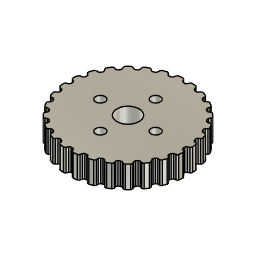
Timing Pulley Motor (Autodesk Fusion 360 design; units mm, degrees)
Autodesk Fusion 360 part; units mm, degrees
note: some values were not read from the file. Set by a fixed rule: which sketch regions a step uses.
(part 1 of 2)
sketch "スケッチ1" plane through (0, 0, 0) normal (0, 0, 1) x (1, 0, 0)
  circle A0 centre (0, 0) radius 4
  line L0 (-4, 0) -> (3, 0)
  line L1 (3, 2.6458) -> (3, -2.6458)
  circle A1 centre (0, 0) radius 20
  dimension "d1" = 8
  dimension "d2" = 7
  dimension "d3" = 40
  constraint coincident A0.centre A1.centre
  constraint coincident A0 L0.start
  constraint horizontal L0
  constraint coincident A0 L1.start
  constraint coincident A0 L1.end
  constraint perpendicular L0 L1
  measures "d1" diameter of A0
  measures "d2" distance of L0.start L0.end
  measures "d3" diameter of A1
extrude "押し出し1" add sketch "スケッチ1" along normal blind 8 contours A0 L1 | A0 L0 L1 | A0 L0 L1 | A1
sketch "スケッチ2" plane through (0, 0, 8) normal (0, 0, 1) x (-1, 0, 0)
  circle A0 centre (0, 0) radius 20
  circle A1 centre (0, 0) radius 22.635
  line L0 (0, 0) -> (22.635, 0)
  line L1 (0, 0) -> (22.0675, 5.0368)
  line L2 (0, 0) -> (20.3934, 9.821)
  line L3 (0, 0) -> (17.6968, 14.1127)
  line L4 (0, 0) -> (14.1127, 17.6968)
  line L5 (0, 0) -> (9.821, 20.3934)
  line L6 (0, 0) -> (5.0368, 22.0675)
  line L7 (0, 0) -> (0, 22.635)
  line L8 (0, 0) -> (-5.0368, 22.0675)
  line L9 (0, 0) -> (-9.821, 20.3934)
  line L10 (0, 0) -> (-14.1127, 17.6968)
  line L11 (0, 0) -> (-17.6968, 14.1127)
  line L12 (0, 0) -> (-20.3934, 9.821)
  line L13 (0, 0) -> (-22.0675, 5.0368)
  line L14 (0, 0) -> (-22.635, 0)
  line L15 (0, 0) -> (-22.0675, -5.0368)
  line L16 (0, 0) -> (-20.3934, -9.821)
  line L17 (0, 0) -> (-17.6968, -14.1127)
  line L18 (0, 0) -> (-14.1127, -17.6968)
  line L19 (0, 0) -> (-9.821, -20.3934)
  line L20 (0, 0) -> (-5.0368, -22.0675)
  line L21 (0, 0) -> (0, -22.635)
  line L22 (0, 0) -> (5.0368, -22.0675)
  line L23 (0, 0) -> (9.821, -20.3934)
  line L24 (0, 0) -> (14.1127, -17.6968)
  line L25 (0, 0) -> (17.6968, -14.1127)
  line L26 (0, 0) -> (20.3934, -9.821)
  line L27 (0, 0) -> (22.0675, -5.0368)
  line L28 (20.5872, -0.8492) -> (21.2144, -1.1417)
  line L29 (20.235, -0.685) -> (21.7353, -0.685) construction
  line L30 (20.5872, 0.8492) -> (21.2144, 1.1417)
  line L31 (20.235, 0.685) -> (21.7353, 0.685) construction
  arc A2 (20.235, -0.2964) -> (20.5872, -0.8492) centre (20.845, -0.2964) ccw
  arc A3 (20.5872, 0.8492) -> (20.235, 0.2964) centre (20.845, 0.2964) ccw
  arc A4 (21.5646, -1.7437) -> (21.2144, -1.1417) centre (20.9566, -1.6945) ccw
  arc A5 (21.2144, 1.1417) -> (21.5646, 1.7437) centre (20.9566, 1.6945) ccw
  arc A6 (21.412, 3.0986) -> (20.9366, 3.6076) centre (20.8082, 3.0112) ccw
  line L32 (20.26, 3.7531) -> (20.9366, 3.6076)
  arc A7 (19.7936, 4.2138) -> (20.26, 3.7531) centre (20.3883, 4.3495) ccw
  arc A8 (19.8821, 5.409) -> (19.6617, 4.7917) centre (20.2564, 4.9274) ccw
  line L33 (19.8821, 5.409) -> (20.4285, 5.8337)
  arc A9 (20.4285, 5.8337) -> (20.6359, 6.4986) centre (20.0541, 6.3153) ccw
  arc A10 (20.1856, 7.7855) -> (19.6089, 8.1759) centre (19.6165, 7.566) ccw
  line L34 (18.9169, 8.1673) -> (19.6089, 8.1759)
  arc A11 (18.3597, 8.5126) -> (18.9169, 8.1673) centre (18.9093, 8.7773) ccw
  arc A12 (18.18, 9.6976) -> (18.1025, 9.0467) centre (18.6521, 9.3113) ccw
  line L35 (18.18, 9.6976) -> (18.6181, 10.2332)
  arc A13 (18.6181, 10.2332) -> (18.6725, 10.9276) centre (18.146, 10.6195) ccw
  arc A14 (17.9471, 12.082) -> (17.2979, 12.3343) centre (17.4411, 11.7414) ccw
  line L36 (16.6252, 12.172) -> (17.2979, 12.3343)
  arc A15 (16.0052, 12.3846) -> (16.6252, 12.172) centre (16.4821, 12.7649) ccw
  arc A16 (15.5662, 13.4999) -> (15.6356, 12.848) centre (16.1125, 13.2284) ccw
  line L37 (15.5662, 13.4999) -> (15.8742, 14.1196)
  arc A17 (15.8742, 14.1196) -> (15.7727, 14.8086) centre (15.328, 14.3911) ccw
  arc A18 (14.8086, 15.7727) -> (14.1196, 15.8742) centre (14.3911, 15.328) ccw
  line L38 (13.4999, 15.5662) -> (14.1196, 15.8742)
  arc A19 (12.848, 15.6356) -> (13.4999, 15.5662) centre (13.2284, 16.1125) ccw
  arc A20 (12.172, 16.6252) -> (12.3846, 16.0052) centre (12.7649, 16.4821) ccw
  line L39 (12.172, 16.6252) -> (12.3343, 17.2979)
  arc A21 (12.3343, 17.2979) -> (12.082, 17.9471) centre (11.7414, 17.4411) ccw
  arc A22 (10.9276, 18.6725) -> (10.2332, 18.6181) centre (10.6195, 18.146) ccw
  line L40 (9.6976, 18.18) -> (10.2332, 18.6181)
  arc A23 (9.0467, 18.1025) -> (9.6976, 18.18) centre (9.3113, 18.6521) ccw
  arc A24 (8.1673, 18.9169) -> (8.5126, 18.3597) centre (8.7773, 18.9093) ccw
  line L41 (8.1673, 18.9169) -> (8.1759, 19.6089)
  arc A25 (8.1759, 19.6089) -> (7.7855, 20.1856) centre (7.566, 19.6165) ccw
  arc A26 (6.4986, 20.6359) -> (5.8337, 20.4285) centre (6.3153, 20.0541) ccw
  line L42 (5.409, 19.8821) -> (5.8337, 20.4285)
  arc A27 (4.7917, 19.6617) -> (5.409, 19.8821) centre (4.9274, 20.2564) ccw
  arc A28 (3.7531, 20.26) -> (4.2138, 19.7936) centre (4.3495, 20.3883) ccw
  line L43 (3.7531, 20.26) -> (3.6076, 20.9366)
  arc A29 (3.6076, 20.9366) -> (3.0986, 21.412) centre (3.0112, 20.8082) ccw
  arc A30 (1.7437, 21.5646) -> (1.1417, 21.2144) centre (1.6945, 20.9566) ccw
  line L44 (0.8492, 20.5872) -> (1.1417, 21.2144)
  arc A31 (0.2964, 20.235) -> (0.8492, 20.5872) centre (0.2964, 20.845) ccw
  arc A32 (-0.8492, 20.5872) -> (-0.2964, 20.235) centre (-0.2964, 20.845) ccw
  line L45 (-0.8492, 20.5872) -> (-1.1417, 21.2144)
  arc A33 (-1.1417, 21.2144) -> (-1.7437, 21.5646) centre (-1.6945, 20.9566) ccw
  arc A34 (-3.0986, 21.412) -> (-3.6076, 20.9366) centre (-3.0112, 20.8082) ccw
  line L46 (-3.7531, 20.26) -> (-3.6076, 20.9366)
  arc A35 (-4.2138, 19.7936) -> (-3.7531, 20.26) centre (-4.3495, 20.3883) ccw
  arc A36 (-5.409, 19.8821) -> (-4.7917, 19.6617) centre (-4.9274, 20.2564) ccw
  line L47 (-5.409, 19.8821) -> (-5.8337, 20.4285)
  arc A37 (-5.8337, 20.4285) -> (-6.4986, 20.6359) centre (-6.3153, 20.0541) ccw
  arc A38 (-7.7855, 20.1856) -> (-8.1759, 19.6089) centre (-7.566, 19.6165) ccw
  line L48 (-8.1673, 18.9169) -> (-8.1759, 19.6089)
  arc A39 (-8.5126, 18.3597) -> (-8.1673, 18.9169) centre (-8.7773, 18.9093) ccw
  arc A40 (-9.6976, 18.18) -> (-9.0467, 18.1025) centre (-9.3113, 18.6521) ccw
  line L49 (-9.6976, 18.18) -> (-10.2332, 18.6181)
  arc A41 (-10.2332, 18.6181) -> (-10.9276, 18.6725) centre (-10.6195, 18.146) ccw
  arc A42 (-12.082, 17.9471) -> (-12.3343, 17.2979) centre (-11.7414, 17.4411) ccw
  line L50 (-12.172, 16.6252) -> (-12.3343, 17.2979)
  arc A43 (-12.3846, 16.0052) -> (-12.172, 16.6252) centre (-12.7649, 16.4821) ccw
  arc A44 (-13.4999, 15.5662) -> (-12.848, 15.6356) centre (-13.2284, 16.1125) ccw
  line L51 (-13.4999, 15.5662) -> (-14.1196, 15.8742)
  arc A45 (-14.1196, 15.8742) -> (-14.8086, 15.7727) centre (-14.3911, 15.328) ccw
  arc A46 (-15.7727, 14.8086) -> (-15.8742, 14.1196) centre (-15.328, 14.3911) ccw
  line L52 (-15.5662, 13.4999) -> (-15.8742, 14.1196)
  arc A47 (-15.6356, 12.848) -> (-15.5662, 13.4999) centre (-16.1125, 13.2284) ccw
  arc A48 (-16.6252, 12.172) -> (-16.0052, 12.3846) centre (-16.4821, 12.7649) ccw
  line L53 (-16.6252, 12.172) -> (-17.2979, 12.3343)
  arc A49 (-17.2979, 12.3343) -> (-17.9471, 12.082) centre (-17.4411, 11.7414) ccw
  arc A50 (-18.6725, 10.9276) -> (-18.6181, 10.2332) centre (-18.146, 10.6195) ccw
  line L54 (-18.18, 9.6976) -> (-18.6181, 10.2332)
  arc A51 (-18.1025, 9.0467) -> (-18.18, 9.6976) centre (-18.6521, 9.3113) ccw
  arc A52 (-18.9169, 8.1673) -> (-18.3597, 8.5126) centre (-18.9093, 8.7773) ccw
  line L55 (-18.9169, 8.1673) -> (-19.6089, 8.1759)
  arc A53 (-19.6089, 8.1759) -> (-20.1856, 7.7855) centre (-19.6165, 7.566) ccw
  arc A54 (-20.6359, 6.4986) -> (-20.4285, 5.8337) centre (-20.0541, 6.3153) ccw
  line L56 (-19.8821, 5.409) -> (-20.4285, 5.8337)
  arc A55 (-19.6617, 4.7917) -> (-19.8821, 5.409) centre (-20.2564, 4.9274) ccw
  arc A56 (-20.26, 3.7531) -> (-19.7936, 4.2138) centre (-20.3883, 4.3495) ccw
  line L57 (-20.26, 3.7531) -> (-20.9366, 3.6076)
  arc A57 (-20.9366, 3.6076) -> (-21.412, 3.0986) centre (-20.8082, 3.0112) ccw
  arc A58 (-21.5646, 1.7437) -> (-21.2144, 1.1417) centre (-20.9566, 1.6945) ccw
  line L58 (-20.5872, 0.8492) -> (-21.2144, 1.1417)
  arc A59 (-20.235, 0.2964) -> (-20.5872, 0.8492) centre (-20.845, 0.2964) ccw
  arc A60 (-20.5872, -0.8492) -> (-20.235, -0.2964) centre (-20.845, -0.2964) ccw
  line L59 (-20.5872, -0.8492) -> (-21.2144, -1.1417)
  arc A61 (-21.2144, -1.1417) -> (-21.5646, -1.7437) centre (-20.9566, -1.6945) ccw
  arc A62 (-21.412, -3.0986) -> (-20.9366, -3.6076) centre (-20.8082, -3.0112) ccw
  line L60 (-20.26, -3.7531) -> (-20.9366, -3.6076)
  arc A63 (-19.7936, -4.2138) -> (-20.26, -3.7531) centre (-20.3883, -4.3495) ccw
  arc A64 (-19.8821, -5.409) -> (-19.6617, -4.7917) centre (-20.2564, -4.9274) ccw
  line L61 (-19.8821, -5.409) -> (-20.4285, -5.8337)
  arc A65 (-20.4285, -5.8337) -> (-20.6359, -6.4986) centre (-20.0541, -6.3153) ccw
  arc A66 (-20.1856, -7.7855) -> (-19.6089, -8.1759) centre (-19.6165, -7.566) ccw
  line L62 (-18.9169, -8.1673) -> (-19.6089, -8.1759)
  arc A67 (-18.3597, -8.5126) -> (-18.9169, -8.1673) centre (-18.9093, -8.7773) ccw
  arc A68 (-18.18, -9.6976) -> (-18.1025, -9.0467) centre (-18.6521, -9.3113) ccw
  line L63 (-18.18, -9.6976) -> (-18.6181, -10.2332)
  arc A69 (-18.6181, -10.2332) -> (-18.6725, -10.9276) centre (-18.146, -10.6195) ccw
  arc A70 (-17.9471, -12.082) -> (-17.2979, -12.3343) centre (-17.4411, -11.7414) ccw
  line L64 (-16.6252, -12.172) -> (-17.2979, -12.3343)
  arc A71 (-16.0052, -12.3846) -> (-16.6252, -12.172) centre (-16.4821, -12.7649) ccw
  arc A72 (-15.5662, -13.4999) -> (-15.6356, -12.848) centre (-16.1125, -13.2284) ccw
  line L65 (-15.5662, -13.4999) -> (-15.8742, -14.1196)
  arc A73 (-15.8742, -14.1196) -> (-15.7727, -14.8086) centre (-15.328, -14.3911) ccw
  arc A74 (-14.8086, -15.7727) -> (-14.1196, -15.8742) centre (-14.3911, -15.328) ccw
  line L66 (-13.4999, -15.5662) -> (-14.1196, -15.8742)
  arc A75 (-12.848, -15.6356) -> (-13.4999, -15.5662) centre (-13.2284, -16.1125) ccw
  arc A76 (-12.172, -16.6252) -> (-12.3846, -16.0052) centre (-12.7649, -16.4821) ccw
  line L67 (-12.172, -16.6252) -> (-12.3343, -17.2979)
  arc A77 (-12.3343, -17.2979) -> (-12.082, -17.9471) centre (-11.7414, -17.4411) ccw
  arc A78 (-10.9276, -18.6725) -> (-10.2332, -18.6181) centre (-10.6195, -18.146) ccw
  line L68 (-9.6976, -18.18) -> (-10.2332, -18.6181)
  arc A79 (-9.0467, -18.1025) -> (-9.6976, -18.18) centre (-9.3113, -18.6521) ccw
  arc A80 (-8.1673, -18.9169) -> (-8.5126, -18.3597) centre (-8.7773, -18.9093) ccw
  line L69 (-8.1673, -18.9169) -> (-8.1759, -19.6089)
  arc A81 (-8.1759, -19.6089) -> (-7.7855, -20.1856) centre (-7.566, -19.6165) ccw
  arc A82 (-6.4986, -20.6359) -> (-5.8337, -20.4285) centre (-6.3153, -20.0541) ccw
  line L70 (-5.409, -19.8821) -> (-5.8337, -20.4285)
  arc A83 (-4.7917, -19.6617) -> (-5.409, -19.8821) centre (-4.9274, -20.2564) ccw
  arc A84 (-3.7531, -20.26) -> (-4.2138, -19.7936) centre (-4.3495, -20.3883) ccw
  line L71 (-3.7531, -20.26) -> (-3.6076, -20.9366)
  arc A85 (-3.6076, -20.9366) -> (-3.0986, -21.412) centre (-3.0112, -20.8082) ccw
  arc A86 (-1.7437, -21.5646) -> (-1.1417, -21.2144) centre (-1.6945, -20.9566) ccw
  line L72 (-0.8492, -20.5872) -> (-1.1417, -21.2144)
  arc A87 (-0.2964, -20.235) -> (-0.8492, -20.5872) centre (-0.2964, -20.845) ccw
  arc A88 (0.8492, -20.5872) -> (0.2964, -20.235) centre (0.2964, -20.845) ccw
  line L73 (0.8492, -20.5872) -> (1.1417, -21.2144)
  arc A89 (1.1417, -21.2144) -> (1.7437, -21.5646) centre (1.6945, -20.9566) ccw
  arc A90 (3.0986, -21.412) -> (3.6076, -20.9366) centre (3.0112, -20.8082) ccw
  line L74 (3.7531, -20.26) -> (3.6076, -20.9366)
  arc A91 (4.2138, -19.7936) -> (3.7531, -20.26) centre (4.3495, -20.3883) ccw
  arc A92 (5.409, -19.8821) -> (4.7917, -19.6617) centre (4.9274, -20.2564) ccw
  line L75 (5.409, -19.8821) -> (5.8337, -20.4285)
  arc A93 (5.8337, -20.4285) -> (6.4986, -20.6359) centre (6.3153, -20.0541) ccw
  arc A94 (7.7855, -20.1856) -> (8.1759, -19.6089) centre (7.566, -19.6165) ccw
  line L76 (8.1673, -18.9169) -> (8.1759, -19.6089)
  arc A95 (8.5126, -18.3597) -> (8.1673, -18.9169) centre (8.7773, -18.9093) ccw
  arc A96 (9.6976, -18.18) -> (9.0467, -18.1025) centre (9.3113, -18.6521) ccw
  line L77 (9.6976, -18.18) -> (10.2332, -18.6181)
  arc A97 (10.2332, -18.6181) -> (10.9276, -18.6725) centre (10.6195, -18.146) ccw
  arc A98 (12.082, -17.9471) -> (12.3343, -17.2979) centre (11.7414, -17.4411) ccw
  line L78 (12.172, -16.6252) -> (12.3343, -17.2979)
  arc A99 (12.3846, -16.0052) -> (12.172, -16.6252) centre (12.7649, -16.4821) ccw
  arc A100 (13.4999, -15.5662) -> (12.848, -15.6356) centre (13.2284, -16.1125) ccw
  line L79 (13.4999, -15.5662) -> (14.1196, -15.8742)
  arc A101 (14.1196, -15.8742) -> (14.8086, -15.7727) centre (14.3911, -15.328) ccw
  arc A102 (15.7727, -14.8086) -> (15.8742, -14.1196) centre (15.328, -14.3911) ccw
  line L80 (15.5662, -13.4999) -> (15.8742, -14.1196)
  arc A103 (15.6356, -12.848) -> (15.5662, -13.4999) centre (16.1125, -13.2284) ccw
  arc A104 (16.6252, -12.172) -> (16.0052, -12.3846) centre (16.4821, -12.7649) ccw
  line L81 (16.6252, -12.172) -> (17.2979, -12.3343)
  arc A105 (17.2979, -12.3343) -> (17.9471, -12.082) centre (17.4411, -11.7414) ccw
  arc A106 (18.6725, -10.9276) -> (18.6181, -10.2332) centre (18.146, -10.6195) ccw
  line L82 (18.18, -9.6976) -> (18.6181, -10.2332)
  arc A107 (18.1025, -9.0467) -> (18.18, -9.6976) centre (18.6521, -9.3113) ccw
  arc A108 (18.9169, -8.1673) -> (18.3597, -8.5126) centre (18.9093, -8.7773) ccw
  line L83 (18.9169, -8.1673) -> (19.6089, -8.1759)
  arc A109 (19.6089, -8.1759) -> (20.1856, -7.7855) centre (19.6165, -7.566) ccw
  arc A110 (20.6359, -6.4986) -> (20.4285, -5.8337) centre (20.0541, -6.3153) ccw
  line L84 (19.8821, -5.409) -> (20.4285, -5.8337)
  arc A111 (19.6617, -4.7917) -> (19.8821, -5.409) centre (20.2564, -4.9274) ccw
  arc A112 (20.26, -3.7531) -> (19.7936, -4.2138) centre (20.3883, -4.3495) ccw
  line L85 (20.26, -3.7531) -> (20.9366, -3.6076)
  arc A113 (20.9366, -3.6076) -> (21.412, -3.0986) centre (20.8082, -3.0112) ccw
  arc A114 (20.235, -0.2964) -> (20.235, 0.2964) centre (0, 0) ccw
  arc A115 (21.412, -3.0986) -> (21.5646, -1.7437) centre (0, 0) ccw
  arc A116 (21.5646, 1.7437) -> (21.412, 3.0986) centre (0, 0) ccw
  arc A117 (19.7936, 4.2138) -> (19.6617, 4.7917) centre (0, 0) ccw
  arc A118 (20.6359, 6.4986) -> (20.1856, 7.7855) centre (0, 0) ccw
  arc A119 (18.3597, 8.5126) -> (18.1025, 9.0467) centre (0, 0) ccw
  arc A120 (18.6725, 10.9276) -> (17.9471, 12.082) centre (0, 0) ccw
  arc A121 (16.0052, 12.3846) -> (15.6356, 12.848) centre (0, 0) ccw
  arc A122 (15.7727, 14.8086) -> (14.8086, 15.7727) centre (0, 0) ccw
  arc A123 (12.848, 15.6356) -> (12.3846, 16.0052) centre (0, 0) ccw
  arc A124 (12.082, 17.9471) -> (10.9276, 18.6725) centre (0, 0) ccw
  arc A125 (9.0467, 18.1025) -> (8.5126, 18.3597) centre (0, 0) ccw
  arc A126 (7.7855, 20.1856) -> (6.4986, 20.6359) centre (0, 0) ccw
  arc A127 (4.7917, 19.6617) -> (4.2138, 19.7936) centre (0, 0) ccw
  arc A128 (3.0986, 21.412) -> (1.7437, 21.5646) centre (0, 0) ccw
  arc A129 (0.2964, 20.235) -> (-0.2964, 20.235) centre (0, 0) ccw
  arc A130 (-1.7437, 21.5646) -> (-3.0986, 21.412) centre (0, 0) ccw
  arc A131 (-4.2138, 19.7936) -> (-4.7917, 19.6617) centre (0, 0) ccw
  arc A132 (-6.4986, 20.6359) -> (-7.7855, 20.1856) centre (0, 0) ccw
  arc A133 (-8.5126, 18.3597) -> (-9.0467, 18.1025) centre (0, 0) ccw
  arc A134 (-10.9276, 18.6725) -> (-12.082, 17.9471) centre (0, 0) ccw
  arc A135 (-12.3846, 16.0052) -> (-12.848, 15.6356) centre (0, 0) ccw
  arc A136 (-14.8086, 15.7727) -> (-15.7727, 14.8086) centre (0, 0) ccw
  arc A137 (-15.6356, 12.848) -> (-16.0052, 12.3846) centre (0, 0) ccw
  arc A138 (-17.9471, 12.082) -> (-18.6725, 10.9276) centre (0, 0) ccw
  arc A139 (-18.1025, 9.0467) -> (-18.3597, 8.5126) centre (0, 0) ccw
  arc A140 (-20.1856, 7.7855) -> (-20.6359, 6.4986) centre (0, 0) ccw
  arc A141 (-19.6617, 4.7917) -> (-19.7936, 4.2138) centre (0, 0) ccw
  arc A142 (-21.412, 3.0986) -> (-21.5646, 1.7437) centre (0, 0) ccw
  arc A143 (-20.235, 0.2964) -> (-20.235, -0.2964) centre (0, 0) ccw
  arc A144 (-21.5646, -1.7437) -> (-21.412, -3.0986) centre (0, 0) ccw
  arc A145 (-19.7936, -4.2138) -> (-19.6617, -4.7917) centre (0, 0) ccw
  arc A146 (-20.6359, -6.4986) -> (-20.1856, -7.7855) centre (0, 0) ccw
  arc A147 (-18.3597, -8.5126) -> (-18.1025, -9.0467) centre (0, 0) ccw
  arc A148 (-18.6725, -10.9276) -> (-17.9471, -12.082) centre (0, 0) ccw
  arc A149 (-16.0052, -12.3846) -> (-15.6356, -12.848) centre (0, 0) ccw
  arc A150 (-15.7727, -14.8086) -> (-14.8086, -15.7727) centre (0, 0) ccw
  arc A151 (-12.848, -15.6356) -> (-12.3846, -16.0052) centre (0, 0) ccw
  arc A152 (-12.082, -17.9471) -> (-10.9276, -18.6725) centre (0, 0) ccw
  arc A153 (-9.0467, -18.1025) -> (-8.5126, -18.3597) centre (0, 0) ccw
  arc A154 (-7.7855, -20.1856) -> (-6.4986, -20.6359) centre (0, 0) ccw
  arc A155 (-4.7917, -19.6617) -> (-4.2138, -19.7936) centre (0, 0) ccw
  arc A156 (-3.0986, -21.412) -> (-1.7437, -21.5646) centre (0, 0) ccw
  arc A157 (-0.2964, -20.235) -> (0.2964, -20.235) centre (0, 0) ccw
  arc A158 (1.7437, -21.5646) -> (3.0986, -21.412) centre (0, 0) ccw
  arc A159 (4.2138, -19.7936) -> (4.7917, -19.6617) centre (0, 0) ccw
  arc A160 (6.4986, -20.6359) -> (7.7855, -20.1856) centre (0, 0) ccw
  arc A161 (8.5126, -18.3597) -> (9.0467, -18.1025) centre (0, 0) ccw
  arc A162 (10.9276, -18.6725) -> (12.082, -17.9471) centre (0, 0) ccw
  arc A163 (12.3846, -16.0052) -> (12.848, -15.6356) centre (0, 0) ccw
  arc A164 (14.8086, -15.7727) -> (15.7727, -14.8086) centre (0, 0) ccw
  arc A165 (15.6356, -12.848) -> (16.0052, -12.3846) centre (0, 0) ccw
  arc A166 (17.9471, -12.082) -> (18.6725, -10.9276) centre (0, 0) ccw
  arc A167 (18.1025, -9.0467) -> (18.3597, -8.5126) centre (0, 0) ccw
  arc A168 (20.1856, -7.7855) -> (20.6359, -6.4986) centre (0, 0) ccw
  arc A169 (19.6617, -4.7917) -> (19.7936, -4.2138) centre (0, 0) ccw
  point P0 (21.5948, -1.3191)
  point P1 (21.5948, 1.3191)
  point P2 (21.0926, -4.8142)
  point P3 (21.0926, 4.8142)
  dimension "d6" = 45.27
  dimension "d8" = 360
  dimension "d17" = 25
  dimension "d18" = 25
  dimension "d19" = 0.61
  dimension "d20" = 0.61
  dimension "d21" = 0.61
  dimension "d22" = 0.61
  dimension "d24" = 360
  dimension "d26" = 360
  constraint coincident A0.centre A1.centre
  constraint coincident A1 L0.end
  constraint horizontal L29
  constraint horizontal L31
  constraint coincident L29.start L28
  constraint tangent L28 A2
  constraint coincident L31.start L30
  constraint tangent L30 A3
  constraint coincident L27 P2
  constraint coincident L1 P3
  constraint tangent L28 A4
  constraint tangent L30 A5
  measures "d6" diameter of A1
  measures "d17" angle of L28 L29
  measures "d18" angle of L30 L31
  measures "d19" radius of A2
  measures "d20" radius of A3
  measures "d21" radius of A4
  measures "d22" radius of A5
extrude "押し出し2" add sketch "スケッチ2" against normal blind 8 contours A0 L0 L27 L28 A2 A4 A112 L85 A113 A114 A115 A169 | A0 L0 L1 L30 A3 A5 A6 L32 A7 A114 A116 A117 | A0 L1 L2 A8 L33 A9 A10 L34 A11 A117 A118 A119 | A0 L26 L27 A108 L83 A109 A110 L84 A111 A167 A168 A169 | A0 L2 L3 A12 L35 A13 A14 L36 A15 A119 A120 A121 | A0 L25 L26 A104 L81 A105 A106 L82 A107 A165 A166 A167 | A0 L3 L4 A16 L37 A17 A18 L38 A19 A121 A122 A123 | A0 L4 L5 A20 L39 A21 A22 L40 A23 A123 A124 A125 | A0 L5 L6 A24 L41 A25 A26 L42 A27 A125 A126 A127 | A0 L6 L7 A28 L43 A29 A30 L44 A31 A127 A128 A129 | A0 L7 L8 A32 L45 A33 A34 L46 A35 A129 A130 A131 | A0 L8 L9 A36 L47 A37 A38 L48 A39 A131 A132 A133 | A0 L9 L10 A40 L49 A41 A42 L50 A43 A133 A134 A135 | A0 L10 L11 A44 L51 A45 A46 L52 A47 A135 A136 A137 | A0 L11 L12 A48 L53 A49 A50 L54 A51 A137 A138 A139 | A0 L12 L13 A52 L55 A53 A54 L56 A55 A139 A140 A141 | A0 L13 L14 A56 L57 A57 A58 L58 A59 A141 A142 A143 | A0 L14 L15 A60 L59 A61 A62 L60 A63 A143 A144 A145 | A0 L15 L16 A64 L61 A65 A66 L62 A67 A145 A146 A147 | A0 L16 L17 A68 L63 A69 A70 L64 A71 A147 A148 A149 | A0 L17 L18 A72 L65 A73 A74 L66 A75 A149 A150 A151 | A0 L18 L19 A76 L67 A77 A78 L68 A79 A151 A152 A153 | A0 L19 L20 A80 L69 A81 A82 L70 A83 A153 A154 A155 | A0 L20 L21 A84 L71 A85 A86 L72 A87 A155 A156 A157 | A0 L21 L22 A88 L73 A89 A90 L74 A91 A157 A158 A159 | A0 L22 L23 A92 L75 A93 A94 L76 A95 A159 A160 A161 | A0 L23 L24 A96 L77 A97 A98 L78 A99 A161 A162 A163 | A0 L24 L25 A100 L79 A101 A102 L80 A103 A163 A164 A165
sketch "スケッチ6" plane through (0, 0, 8) normal (0, 0, 1) x (-1, 0, 0)
  arc A0 (19.6617, -4.7917) -> (19.8821, -5.409) centre (20.2564, -4.9274) ccw
  arc A1 (19.6617, -4.7917) -> (19.7936, -4.2138) centre (0, 0) ccw
  arc A2 (20.26, -3.7531) -> (19.7936, -4.2138) centre (20.3883, -4.3495) ccw
  line L0 (20.26, -3.7531) -> (20.9366, -3.6076)
  arc A3 (20.9366, -3.6076) -> (21.412, -3.0986) centre (20.8082, -3.0112) ccw
  arc A4 (21.412, -3.0986) -> (21.5646, -1.7437) centre (0, 0) ccw
  arc A5 (21.5646, -1.7437) -> (21.2144, -1.1417) centre (20.9566, -1.6945) ccw
  line L1 (21.2144, -1.1417) -> (20.5872, -0.8492)
  arc A6 (20.235, -0.2964) -> (20.5872, -0.8492) centre (20.845, -0.2964) ccw
  arc A7 (20.235, -0.2964) -> (20.235, 0.2964) centre (0, 0) ccw
  arc A8 (20.5872, 0.8492) -> (20.235, 0.2964) centre (20.845, 0.2964) ccw
  line L2 (20.5872, 0.8492) -> (21.2144, 1.1417)
  arc A9 (21.2144, 1.1417) -> (21.5646, 1.7437) centre (20.9566, 1.6945) ccw
  arc A10 (21.5646, 1.7437) -> (21.412, 3.0986) centre (0, 0) ccw
  arc A11 (21.412, 3.0986) -> (20.9366, 3.6076) centre (20.8082, 3.0112) ccw
  line L3 (20.9366, 3.6076) -> (20.26, 3.7531)
  arc A12 (19.7936, 4.2138) -> (20.26, 3.7531) centre (20.3883, 4.3495) ccw
  arc A13 (19.7936, 4.2138) -> (19.6617, 4.7917) centre (0, 0) ccw
  arc A14 (19.8821, 5.409) -> (19.6617, 4.7917) centre (20.2564, 4.9274) ccw
  line L4 (19.8821, 5.409) -> (20.4285, 5.8337)
  arc A15 (20.4285, 5.8337) -> (20.6359, 6.4986) centre (20.0541, 6.3153) ccw
  arc A16 (20.6359, 6.4986) -> (20.1856, 7.7855) centre (0, 0) ccw
  arc A17 (20.1856, 7.7855) -> (19.6089, 8.1759) centre (19.6165, 7.566) ccw
  line L5 (19.6089, 8.1759) -> (18.9169, 8.1673)
  arc A18 (18.3597, 8.5126) -> (18.9169, 8.1673) centre (18.9093, 8.7773) ccw
  arc A19 (18.3597, 8.5126) -> (18.1025, 9.0467) centre (0, 0) ccw
  arc A20 (18.18, 9.6976) -> (18.1025, 9.0467) centre (18.6521, 9.3113) ccw
  line L6 (18.18, 9.6976) -> (18.6181, 10.2332)
  arc A21 (18.6181, 10.2332) -> (18.6725, 10.9276) centre (18.146, 10.6195) ccw
  arc A22 (18.6725, 10.9276) -> (17.9471, 12.082) centre (0, 0) ccw
  arc A23 (17.9471, 12.082) -> (17.2979, 12.3343) centre (17.4411, 11.7414) ccw
  line L7 (17.2979, 12.3343) -> (16.6252, 12.172)
  arc A24 (16.0052, 12.3846) -> (16.6252, 12.172) centre (16.4821, 12.7649) ccw
  arc A25 (16.0052, 12.3846) -> (15.6356, 12.848) centre (0, 0) ccw
  arc A26 (15.5662, 13.4999) -> (15.6356, 12.848) centre (16.1125, 13.2284) ccw
  line L8 (15.5662, 13.4999) -> (15.8742, 14.1196)
  arc A27 (15.8742, 14.1196) -> (15.7727, 14.8086) centre (15.328, 14.3911) ccw
  arc A28 (15.7727, 14.8086) -> (14.8086, 15.7727) centre (0, 0) ccw
  arc A29 (14.8086, 15.7727) -> (14.1196, 15.8742) centre (14.3911, 15.328) ccw
  line L9 (14.1196, 15.8742) -> (13.4999, 15.5662)
  arc A30 (12.848, 15.6356) -> (13.4999, 15.5662) centre (13.2284, 16.1125) ccw
  arc A31 (12.848, 15.6356) -> (12.3846, 16.0052) centre (0, 0) ccw
  arc A32 (12.172, 16.6252) -> (12.3846, 16.0052) centre (12.7649, 16.4821) ccw
  line L10 (12.172, 16.6252) -> (12.3343, 17.2979)
  arc A33 (12.3343, 17.2979) -> (12.082, 17.9471) centre (11.7414, 17.4411) ccw
  arc A34 (12.082, 17.9471) -> (10.9276, 18.6725) centre (0, 0) ccw
  arc A35 (10.9276, 18.6725) -> (10.2332, 18.6181) centre (10.6195, 18.146) ccw
  line L11 (10.2332, 18.6181) -> (9.6976, 18.18)
  arc A36 (9.0467, 18.1025) -> (9.6976, 18.18) centre (9.3113, 18.6521) ccw
  arc A37 (9.0467, 18.1025) -> (8.5126, 18.3597) centre (0, 0) ccw
  arc A38 (8.1673, 18.9169) -> (8.5126, 18.3597) centre (8.7773, 18.9093) ccw
  line L12 (8.1673, 18.9169) -> (8.1759, 19.6089)
  arc A39 (8.1759, 19.6089) -> (7.7855, 20.1856) centre (7.566, 19.6165) ccw
  arc A40 (7.7855, 20.1856) -> (6.4986, 20.6359) centre (0, 0) ccw
  arc A41 (6.4986, 20.6359) -> (5.8337, 20.4285) centre (6.3153, 20.0541) ccw
  line L13 (5.8337, 20.4285) -> (5.409, 19.8821)
  arc A42 (4.7917, 19.6617) -> (5.409, 19.8821) centre (4.9274, 20.2564) ccw
  arc A43 (4.7917, 19.6617) -> (4.2138, 19.7936) centre (0, 0) ccw
  arc A44 (3.7531, 20.26) -> (4.2138, 19.7936) centre (4.3495, 20.3883) ccw
  line L14 (3.7531, 20.26) -> (3.6076, 20.9366)
  arc A45 (3.6076, 20.9366) -> (3.0986, 21.412) centre (3.0112, 20.8082) ccw
  arc A46 (3.0986, 21.412) -> (1.7437, 21.5646) centre (0, 0) ccw
  arc A47 (1.7437, 21.5646) -> (1.1417, 21.2144) centre (1.6945, 20.9566) ccw
  line L15 (1.1417, 21.2144) -> (0.8492, 20.5872)
  arc A48 (0.2964, 20.235) -> (0.8492, 20.5872) centre (0.2964, 20.845) ccw
  arc A49 (0.2964, 20.235) -> (-0.2964, 20.235) centre (0, 0) ccw
  arc A50 (-0.8492, 20.5872) -> (-0.2964, 20.235) centre (-0.2964, 20.845) ccw
  line L16 (-0.8492, 20.5872) -> (-1.1417, 21.2144)
  arc A51 (-1.1417, 21.2144) -> (-1.7437, 21.5646) centre (-1.6945, 20.9566) ccw
  arc A52 (-1.7437, 21.5646) -> (-3.0986, 21.412) centre (0, 0) ccw
  arc A53 (-3.0986, 21.412) -> (-3.6076, 20.9366) centre (-3.0112, 20.8082) ccw
  line L17 (-3.6076, 20.9366) -> (-3.7531, 20.26)
  arc A54 (-4.2138, 19.7936) -> (-3.7531, 20.26) centre (-4.3495, 20.3883) ccw
  arc A55 (-4.2138, 19.7936) -> (-4.7917, 19.6617) centre (0, 0) ccw
  arc A56 (-5.409, 19.8821) -> (-4.7917, 19.6617) centre (-4.9274, 20.2564) ccw
  line L18 (-5.409, 19.8821) -> (-5.8337, 20.4285)
  arc A57 (-5.8337, 20.4285) -> (-6.4986, 20.6359) centre (-6.3153, 20.0541) ccw
  arc A58 (-6.4986, 20.6359) -> (-7.7855, 20.1856) centre (0, 0) ccw
  arc A59 (-7.7855, 20.1856) -> (-8.1759, 19.6089) centre (-7.566, 19.6165) ccw
  line L19 (-8.1759, 19.6089) -> (-8.1673, 18.9169)
  arc A60 (-8.5126, 18.3597) -> (-8.1673, 18.9169) centre (-8.7773, 18.9093) ccw
  arc A61 (-8.5126, 18.3597) -> (-9.0467, 18.1025) centre (0, 0) ccw
  arc A62 (-9.6976, 18.18) -> (-9.0467, 18.1025) centre (-9.3113, 18.6521) ccw
  line L20 (-9.6976, 18.18) -> (-10.2332, 18.6181)
  arc A63 (-10.2332, 18.6181) -> (-10.9276, 18.6725) centre (-10.6195, 18.146) ccw
  arc A64 (-10.9276, 18.6725) -> (-12.082, 17.9471) centre (0, 0) ccw
  arc A65 (-12.082, 17.9471) -> (-12.3343, 17.2979) centre (-11.7414, 17.4411) ccw
  line L21 (-12.3343, 17.2979) -> (-12.172, 16.6252)
  arc A66 (-12.3846, 16.0052) -> (-12.172, 16.6252) centre (-12.7649, 16.4821) ccw
  arc A67 (-12.3846, 16.0052) -> (-12.848, 15.6356) centre (0, 0) ccw
  arc A68 (-13.4999, 15.5662) -> (-12.848, 15.6356) centre (-13.2284, 16.1125) ccw
  line L22 (-13.4999, 15.5662) -> (-14.1196, 15.8742)
  arc A69 (-14.1196, 15.8742) -> (-14.8086, 15.7727) centre (-14.3911, 15.328) ccw
  arc A70 (-14.8086, 15.7727) -> (-15.7727, 14.8086) centre (0, 0) ccw
  arc A71 (-15.7727, 14.8086) -> (-15.8742, 14.1196) centre (-15.328, 14.3911) ccw
  line L23 (-15.8742, 14.1196) -> (-15.5662, 13.4999)
  arc A72 (-15.6356, 12.848) -> (-15.5662, 13.4999) centre (-16.1125, 13.2284) ccw
  arc A73 (-15.6356, 12.848) -> (-16.0052, 12.3846) centre (0, 0) ccw
  arc A74 (-16.6252, 12.172) -> (-16.0052, 12.3846) centre (-16.4821, 12.7649) ccw
  line L24 (-16.6252, 12.172) -> (-17.2979, 12.3343)
  arc A75 (-17.2979, 12.3343) -> (-17.9471, 12.082) centre (-17.4411, 11.7414) ccw
  arc A76 (-17.9471, 12.082) -> (-18.6725, 10.9276) centre (0, 0) ccw
  arc A77 (-18.6725, 10.9276) -> (-18.6181, 10.2332) centre (-18.146, 10.6195) ccw
  line L25 (-18.6181, 10.2332) -> (-18.18, 9.6976)
  arc A78 (-18.1025, 9.0467) -> (-18.18, 9.6976) centre (-18.6521, 9.3113) ccw
  arc A79 (-18.1025, 9.0467) -> (-18.3597, 8.5126) centre (0, 0) ccw
  arc A80 (-18.9169, 8.1673) -> (-18.3597, 8.5126) centre (-18.9093, 8.7773) ccw
  line L26 (-18.9169, 8.1673) -> (-19.6089, 8.1759)
  arc A81 (-19.6089, 8.1759) -> (-20.1856, 7.7855) centre (-19.6165, 7.566) ccw
  arc A82 (-20.1856, 7.7855) -> (-20.6359, 6.4986) centre (0, 0) ccw
  arc A83 (-20.6359, 6.4986) -> (-20.4285, 5.8337) centre (-20.0541, 6.3153) ccw
  line L27 (-20.4285, 5.8337) -> (-19.8821, 5.409)
  arc A84 (-19.6617, 4.7917) -> (-19.8821, 5.409) centre (-20.2564, 4.9274) ccw
  arc A85 (-19.6617, 4.7917) -> (-19.7936, 4.2138) centre (0, 0) ccw
  arc A86 (-20.26, 3.7531) -> (-19.7936, 4.2138) centre (-20.3883, 4.3495) ccw
  line L28 (-20.26, 3.7531) -> (-20.9366, 3.6076)
  arc A87 (-20.9366, 3.6076) -> (-21.412, 3.0986) centre (-20.8082, 3.0112) ccw
  arc A88 (-21.412, 3.0986) -> (-21.5646, 1.7437) centre (0, 0) ccw
  arc A89 (-21.5646, 1.7437) -> (-21.2144, 1.1417) centre (-20.9566, 1.6945) ccw
  line L29 (-21.2144, 1.1417) -> (-20.5872, 0.8492)
  arc A90 (-20.235, 0.2964) -> (-20.5872, 0.8492) centre (-20.845, 0.2964) ccw
  arc A91 (-20.235, 0.2964) -> (-20.235, -0.2964) centre (0, 0) ccw
  arc A92 (-20.5872, -0.8492) -> (-20.235, -0.2964) centre (-20.845, -0.2964) ccw
  line L30 (-20.5872, -0.8492) -> (-21.2144, -1.1417)
  arc A93 (-21.2144, -1.1417) -> (-21.5646, -1.7437) centre (-20.9566, -1.6945) ccw
  arc A94 (-21.5646, -1.7437) -> (-21.412, -3.0986) centre (0, 0) ccw
  arc A95 (-21.412, -3.0986) -> (-20.9366, -3.6076) centre (-20.8082, -3.0112) ccw
  line L31 (-20.9366, -3.6076) -> (-20.26, -3.7531)
  arc A96 (-19.7936, -4.2138) -> (-20.26, -3.7531) centre (-20.3883, -4.3495) ccw
  arc A97 (-19.7936, -4.2138) -> (-19.6617, -4.7917) centre (0, 0) ccw
  arc A98 (-19.8821, -5.409) -> (-19.6617, -4.7917) centre (-20.2564, -4.9274) ccw
  line L32 (-19.8821, -5.409) -> (-20.4285, -5.8337)
  arc A99 (-20.4285, -5.8337) -> (-20.6359, -6.4986) centre (-20.0541, -6.3153) ccw
  arc A100 (-20.6359, -6.4986) -> (-20.1856, -7.7855) centre (0, 0) ccw
  arc A101 (-20.1856, -7.7855) -> (-19.6089, -8.1759) centre (-19.6165, -7.566) ccw
  line L33 (-19.6089, -8.1759) -> (-18.9169, -8.1673)
  arc A102 (-18.3597, -8.5126) -> (-18.9169, -8.1673) centre (-18.9093, -8.7773) ccw
  arc A103 (-18.3597, -8.5126) -> (-18.1025, -9.0467) centre (0, 0) ccw
  arc A104 (-18.18, -9.6976) -> (-18.1025, -9.0467) centre (-18.6521, -9.3113) ccw
  line L34 (-18.18, -9.6976) -> (-18.6181, -10.2332)
  arc A105 (-18.6181, -10.2332) -> (-18.6725, -10.9276) centre (-18.146, -10.6195) ccw
  arc A106 (-18.6725, -10.9276) -> (-17.9471, -12.082) centre (0, 0) ccw
  arc A107 (-17.9471, -12.082) -> (-17.2979, -12.3343) centre (-17.4411, -11.7414) ccw
  line L35 (-17.2979, -12.3343) -> (-16.6252, -12.172)
  arc A108 (-16.0052, -12.3846) -> (-16.6252, -12.172) centre (-16.4821, -12.7649) ccw
  arc A109 (-16.0052, -12.3846) -> (-15.6356, -12.848) centre (0, 0) ccw
  arc A110 (-15.5662, -13.4999) -> (-15.6356, -12.848) centre (-16.1125, -13.2284) ccw
  line L36 (-15.5662, -13.4999) -> (-15.8742, -14.1196)
  arc A111 (-15.8742, -14.1196) -> (-15.7727, -14.8086) centre (-15.328, -14.3911) ccw
  arc A112 (-15.7727, -14.8086) -> (-14.8086, -15.7727) centre (0, 0) ccw
  arc A113 (-14.8086, -15.7727) -> (-14.1196, -15.8742) centre (-14.3911, -15.328) ccw
  line L37 (-14.1196, -15.8742) -> (-13.4999, -15.5662)
  arc A114 (-12.848, -15.6356) -> (-13.4999, -15.5662) centre (-13.2284, -16.1125) ccw
  arc A115 (-12.848, -15.6356) -> (-12.3846, -16.0052) centre (0, 0) ccw
  arc A116 (-12.172, -16.6252) -> (-12.3846, -16.0052) centre (-12.7649, -16.4821) ccw
  line L38 (-12.172, -16.6252) -> (-12.3343, -17.2979)
  arc A117 (-12.3343, -17.2979) -> (-12.082, -17.9471) centre (-11.7414, -17.4411) ccw
  arc A118 (-12.082, -17.9471) -> (-10.9276, -18.6725) centre (0, 0) ccw
  arc A119 (-10.9276, -18.6725) -> (-10.2332, -18.6181) centre (-10.6195, -18.146) ccw
  line L39 (-10.2332, -18.6181) -> (-9.6976, -18.18)
  arc A120 (-9.0467, -18.1025) -> (-9.6976, -18.18) centre (-9.3113, -18.6521) ccw
  arc A121 (-9.0467, -18.1025) -> (-8.5126, -18.3597) centre (0, 0) ccw
  arc A122 (-8.1673, -18.9169) -> (-8.5126, -18.3597) centre (-8.7773, -18.9093) ccw
  line L40 (-8.1673, -18.9169) -> (-8.1759, -19.6089)
  arc A123 (-8.1759, -19.6089) -> (-7.7855, -20.1856) centre (-7.566, -19.6165) ccw
  arc A124 (-7.7855, -20.1856) -> (-6.4986, -20.6359) centre (0, 0) ccw
  arc A125 (-6.4986, -20.6359) -> (-5.8337, -20.4285) centre (-6.3153, -20.0541) ccw
  line L41 (-5.8337, -20.4285) -> (-5.409, -19.8821)
  arc A126 (-4.7917, -19.6617) -> (-5.409, -19.8821) centre (-4.9274, -20.2564) ccw
  arc A127 (-4.7917, -19.6617) -> (-4.2138, -19.7936) centre (0, 0) ccw
  arc A128 (-3.7531, -20.26) -> (-4.2138, -19.7936) centre (-4.3495, -20.3883) ccw
  line L42 (-3.7531, -20.26) -> (-3.6076, -20.9366)
  arc A129 (-3.6076, -20.9366) -> (-3.0986, -21.412) centre (-3.0112, -20.8082) ccw
  arc A130 (-3.0986, -21.412) -> (-1.7437, -21.5646) centre (0, 0) ccw
  arc A131 (-1.7437, -21.5646) -> (-1.1417, -21.2144) centre (-1.6945, -20.9566) ccw
  line L43 (-1.1417, -21.2144) -> (-0.8492, -20.5872)
  arc A132 (-0.2964, -20.235) -> (-0.8492, -20.5872) centre (-0.2964, -20.845) ccw
  arc A133 (-0.2964, -20.235) -> (0.2964, -20.235) centre (0, 0) ccw
  arc A134 (0.8492, -20.5872) -> (0.2964, -20.235) centre (0.2964, -20.845) ccw
  line L44 (0.8492, -20.5872) -> (1.1417, -21.2144)
  arc A135 (1.1417, -21.2144) -> (1.7437, -21.5646) centre (1.6945, -20.9566) ccw
  arc A136 (1.7437, -21.5646) -> (3.0986, -21.412) centre (0, 0) ccw
  arc A137 (3.0986, -21.412) -> (3.6076, -20.9366) centre (3.0112, -20.8082) ccw
  line L45 (3.6076, -20.9366) -> (3.7531, -20.26)
  arc A138 (4.2138, -19.7936) -> (3.7531, -20.26) centre (4.3495, -20.3883) ccw
  arc A139 (4.2138, -19.7936) -> (4.7917, -19.6617) centre (0, 0) ccw
  arc A140 (5.409, -19.8821) -> (4.7917, -19.6617) centre (4.9274, -20.2564) ccw
  line L46 (5.409, -19.8821) -> (5.8337, -20.4285)
  arc A141 (5.8337, -20.4285) -> (6.4986, -20.6359) centre (6.3153, -20.0541) ccw
  arc A142 (6.4986, -20.6359) -> (7.7855, -20.1856) centre (0, 0) ccw
  arc A143 (7.7855, -20.1856) -> (8.1759, -19.6089) centre (7.566, -19.6165) ccw
  line L47 (8.1759, -19.6089) -> (8.1673, -18.9169)
  arc A144 (8.5126, -18.3597) -> (8.1673, -18.9169) centre (8.7773, -18.9093) ccw
  arc A145 (8.5126, -18.3597) -> (9.0467, -18.1025) centre (0, 0) ccw
  arc A146 (9.6976, -18.18) -> (9.0467, -18.1025) centre (9.3113, -18.6521) ccw
  line L48 (9.6976, -18.18) -> (10.2332, -18.6181)
  arc A147 (10.2332, -18.6181) -> (10.9276, -18.6725) centre (10.6195, -18.146) ccw
  arc A148 (10.9276, -18.6725) -> (12.082, -17.9471) centre (0, 0) ccw
  arc A149 (12.082, -17.9471) -> (12.3343, -17.2979) centre (11.7414, -17.4411) ccw
  line L49 (12.3343, -17.2979) -> (12.172, -16.6252)
  arc A150 (12.3846, -16.0052) -> (12.172, -16.6252) centre (12.7649, -16.4821) ccw
  arc A151 (12.3846, -16.0052) -> (12.848, -15.6356) centre (0, 0) ccw
  arc A152 (13.4999, -15.5662) -> (12.848, -15.6356) centre (13.2284, -16.1125) ccw
  line L50 (13.4999, -15.5662) -> (14.1196, -15.8742)
  arc A153 (14.1196, -15.8742) -> (14.8086, -15.7727) centre (14.3911, -15.328) ccw
  arc A154 (14.8086, -15.7727) -> (15.7727, -14.8086) centre (0, 0) ccw
  arc A155 (15.7727, -14.8086) -> (15.8742, -14.1196) centre (15.328, -14.3911) ccw
  line L51 (15.8742, -14.1196) -> (15.5662, -13.4999)
  arc A156 (15.6356, -12.848) -> (15.5662, -13.4999) centre (16.1125, -13.2284) ccw
  arc A157 (15.6356, -12.848) -> (16.0052, -12.3846) centre (0, 0) ccw
  arc A158 (16.6252, -12.172) -> (16.0052, -12.3846) centre (16.4821, -12.7649) ccw
  line L52 (16.6252, -12.172) -> (17.2979, -12.3343)
  arc A159 (17.2979, -12.3343) -> (17.9471, -12.082) centre (17.4411, -11.7414) ccw
  arc A160 (17.9471, -12.082) -> (18.6725, -10.9276) centre (0, 0) ccw
  arc A161 (18.6725, -10.9276) -> (18.6181, -10.2332) centre (18.146, -10.6195) ccw
  line L53 (18.6181, -10.2332) -> (18.18, -9.6976)
  arc A162 (18.1025, -9.0467) -> (18.18, -9.6976) centre (18.6521, -9.3113) ccw
  arc A163 (18.1025, -9.0467) -> (18.3597, -8.5126) centre (0, 0) ccw
  arc A164 (18.9169, -8.1673) -> (18.3597, -8.5126) centre (18.9093, -8.7773) ccw
  line L54 (18.9169, -8.1673) -> (19.6089, -8.1759)
  arc A165 (19.6089, -8.1759) -> (20.1856, -7.7855) centre (19.6165, -7.566) ccw
  arc A166 (20.1856, -7.7855) -> (20.6359, -6.4986) centre (0, 0) ccw
  arc A167 (20.6359, -6.4986) -> (20.4285, -5.8337) centre (20.0541, -6.3153) ccw
  line L55 (20.4285, -5.8337) -> (19.8821, -5.409)
  circle A168 centre (0, 0) radius 12.5
  line L56 (0, 0) -> (-10, 0)
  circle A169 centre (-10, 0) radius 1
  circle A170 centre (-7.0711, -7.0711) radius 1
  circle A171 centre (0, -10) radius 1
  circle A172 centre (7.0711, -7.0711) radius 1
  circle A173 centre (10, 0) radius 1
  circle A174 centre (7.0711, 7.0711) radius 1
  circle A175 centre (0, 10) radius 1
  circle A176 centre (-7.0711, 7.0711) radius 1
  dimension "d51" = 25
  dimension "d52" = 10
  dimension "d53" = 2
  dimension "d55" = 360
  constraint coincident A1.centre A4.centre
  constraint horizontal L56
  constraint coincident L56.end A169.centre
  measures "d51" diameter of A168
  measures "d52" distance of A1.centre L56.end
  measures "d53" diameter of A169